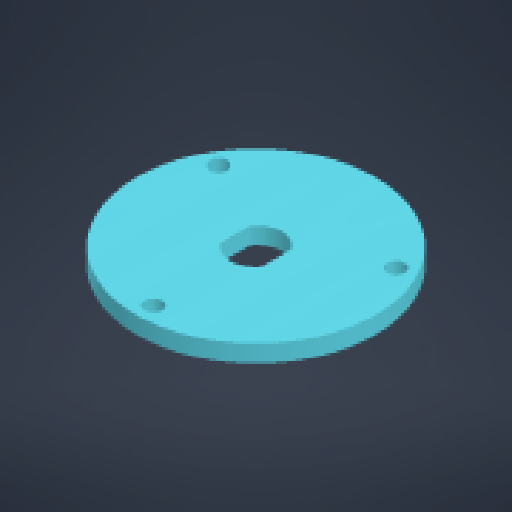
# Autodesk Inventor part: tibea_vodilo_steel
Saved by Autodesk Inventor 2026 (Build 300175000, 175)
## iProperties
Created: 2026-04-25
Part Number: tibea_vodilo_steel
Material: Сталь 09Г2С
Document SubType Name: Modeling
Designer: user
Density: 7.85 g/cm^3
Appearance: Серо-синий
Mass: 113.946 g
Surface Area: 85.1288 cm^2
Volume: 14.5154 cm^3
Author: user
Autodesk Inventor part; units mm, degrees
ref_plane "YZ Plane" through (0, 0, 0) normal (1, 0, 0) x (0, 1, 0)
ref_plane "XZ Plane" through (0, 0, 0) normal (0, 1, 0) x (-1, 0, 0)
ref_plane "XY Plane" through (0, 0, 0) normal (0, 0, 1) x (1, 0, 0)
sketch "Эскиз1" plane through (0, 0, 0) normal (0, 1, 0) x (-1, 0, 0)
  line L0 (48.4444, -57.1419) -> (48.4444, -48.1419) projected
  arc A0 (60.4444, -48.1419) -> (48.4444, -48.1419) centre (54.4444, -52.6419) ccw projected
  line L1 (60.4444, -48.1419) -> (60.4444, -57.1419) projected
  arc A1 (48.4444, -57.1419) -> (60.4444, -57.1419) centre (54.4444, -52.6419) ccw projected
  circle A2 centre (54.4444, -52.6419) radius 30 construction
  circle A3 centre (54.4444, -52.6419) radius 35
  circle A4 centre (28.4636, -67.6419) radius 2.55
  circle A5 centre (54.4444, -52.6419) radius 30 construction
  circle A6 centre (80.4251, -67.6419) radius 2.55
  circle A7 centre (54.4444, -52.6419) radius 30 construction
  circle A8 centre (54.4444, -22.6419) radius 2.55
  point P0 (0, 0)
  point P1 (109.6501, -75.8137)
  dimension "d5" = 60
  dimension "d4" = 70
  dimension "d6" = 5.1
  dimension "d9" = 360
  constraints: 4 centre point, 2 coincident, 2 vertical alignment, 21 other
  measures "d4" diameter of A3
  measures "d6" diameter of A4
extrude "Выдавливание1" add sketch "Эскиз1" along normal blind 4
equation "\"tolerance_plazma\" = 0.1"
equation "\"thickness_steel\" = 3"
equation "\"d_main_screw_holes\" = 6.1"
equation "\"thickness_profile_tibea\" = 3"
equation "\"thickness_profile_femur\" = 3"
equation "\"hight_shaft_shift\" = 37"
equation "\"width_shaft_shift\" = 35"
equation "\"width_flattened_surface\" = 12"
